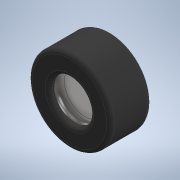
# Autodesk Inventor part: WheelDraft
Saved by Autodesk Inventor 2021 (Build 250183000, 183)
## iProperties
Created: 2021-03-06
Part Number: WheelDraft
Material: Generic
Document SubType Name: Modeling
Designer: M3rob
Density: 1 g/cm^3
Appearance: Default
Author: M3rob
Autodesk Inventor part; units mm, degrees
ref_plane "YZ Plane" through (0, 0, 0) normal (1, 0, 0) x (0, 1, 0)
ref_plane "XZ Plane" through (0, 0, 0) normal (0, 1, 0) x (-1, 0, 0)
ref_plane "XY Plane" through (0, 0, 0) normal (0, 0, 1) x (1, 0, 0)
sketch "Sketch1" plane through (0, 0, 0) normal (1, 0, 0) x (0, 1, 0)
  line L0 (101.6, 50.8) -> (50.8, 50.8)
  line L1 (50.8, 50.8) -> (50.8, 12.7)
  line L2 (101.6, -50.8) -> (101.6, 50.8)
  line L3 (0, 12.7) -> (50.8, 12.7)
  line L4 (0, 12.7) -> (0, -50.8)
  line L5 (0, -50.8) -> (101.6, -50.8)
  arc A0 (50.8, 12.7) -> (50.8, 38.1) centre (50.8, 25.4) ccw
  point P0 (0, 0)
  point P1 (101.6, 0)
  dimension "d0" = 101.6
  dimension "d1" = 101.6
  dimension "d2" = 50.8
  dimension "d3" = 38.1
  dimension "d6" = 25.4
  constraints: 13 end point, 2 parallel, 2 point on circle, 2 point on line, 1 centre point, 1 horizontal, 1 horizontal alignment, 1 midpoint, 1 perpendicular, 1 tangent, 1 vertical
  measures "d0" distance between parallel lines of L4 L2
  measures "d1" distance of L2.start L0.start
  measures "d2" distance of L3.start L1.end
  measures "d3" distance of L0.end L1.end
  measures "d6" distance of L1.end A0.end
revolve "Revolution1" add sketch "Sketch1" angle 360 about axis through (0, 0, 12.7) along (0, 0, -1) contours L2 L5 L4 L3 A0 L1 L0
fillet "Fillet1" radius 9.5377 4 edges at (0, -101.6, 50.8) (0, -50.8, 50.8) (0, -50.8, 12.7) (0, -101.6, -50.8)
equation "\"d1\" = d0"
body "Solid1"
